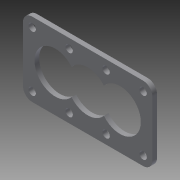
# Autodesk Inventor part: HW 8 Part 5
Saved by Autodesk Inventor 2015 (Build 190159000, 159)
## iProperties
Created: 2016-03-08
Part Number: HW 8 Part 5
Material: Generic
Document SubType Name: Modeling
Designer: Melissa
Density: 1 g/cm^3
Appearance: Default
Author: Melissa
Autodesk Inventor part; units mm, degrees
ref_plane "YZ Plane" through (0, 0, 0) normal (1, 0, 0) x (0, 1, 0)
ref_plane "XZ Plane" through (0, 0, 0) normal (0, 1, 0) x (-1, 0, 0)
ref_plane "XY Plane" through (0, 0, 0) normal (0, 0, 1) x (1, 0, 0)
sketch "Sketch1" plane through (0, 0, 0) normal (0, 0, 1) x (1, 0, 0)
  line L0 (12.7, 0) -> (165.1, 0)
  line L1 (177.8, 12.7) -> (177.8, 88.9)
  line L2 (165.1, 101.6) -> (12.7, 101.6)
  line L3 (0, 88.9) -> (0, 12.7)
  arc A0 (12.7, 101.6) -> (0, 88.9) centre (12.7, 88.9) ccw
  arc A1 (0, 12.7) -> (12.7, 0) centre (12.7, 12.7) ccw
  arc A2 (165.1, 0) -> (177.8, 12.7) centre (165.1, 12.7) ccw
  arc A3 (177.8, 88.9) -> (165.1, 101.6) centre (165.1, 88.9) ccw
  circle A4 centre (12.7, 88.9) radius 5.08
  circle A5 centre (165.1, 88.9) radius 5.08
  circle A6 centre (165.1, 12.7) radius 5.08
  circle A7 centre (12.7, 12.7) radius 5.08
  circle A8 centre (63.5, 88.9) radius 5.08
  circle A9 centre (114.3, 88.9) radius 5.08
  circle A10 centre (63.5, 12.7) radius 5.08
  circle A11 centre (114.3, 12.7) radius 5.08
  arc A12 (111.125, 32.8395) -> (111.125, 68.7605) centre (133.35, 50.8) ccw
  arc A13 (66.675, 68.7605) -> (66.675, 32.8395) centre (44.45, 50.8) ccw
  arc A14 (66.675, 32.8395) -> (111.125, 32.8395) centre (88.9, 50.8) ccw
  arc A15 (111.125, 68.7605) -> (66.675, 68.7605) centre (88.9, 50.8) ccw
  point P0 (0, 0)
  point P1 (177.8, 0)
  point P2 (0, 101.6)
  dimension "d0" = 101.6
  dimension "d1" = 177.8
  dimension "d2" = 12.7
  dimension "d3" = 10.16
  dimension "d4" = 10.16
  dimension "d15" = 50.8
  dimension "d17" = 50.8
  dimension "d18" = 88.9
  dimension "d19" = 57.15
  dimension "d20" = 44.45
  dimension "d21" = 57.15
  dimension "d22" = 44.45
  constraints: 16 centre point, 16 point on circle, 8 end point, 8 tangent, 6 point on line, 4 coincident, 3 equal radius, 2 parallel, 1 horizontal, 1 perpendicular
  measures "d0" distance of point (0, 101.6) point (0, 0)
  measures "d1" distance of point (0, 0) point (177.8, 0)
  measures "d2" radius of A0
  measures "d3" diameter of A4
  measures "d4" diameter of A5
  measures "d15" distance of A10.centre A7.centre
  measures "d17" distance from line of A14.centre L2
  measures "d18" distance from line of L1 A14.centre
  measures "d19" diameter of A12
  measures "d20" distance of A12.centre A14.centre
  measures "d21" diameter of A13
  measures "d22" distance of A14.centre A13.centre
extrude "Extrusion1" add sketch "Sketch1" along normal blind 6.35
body "Solid1"
